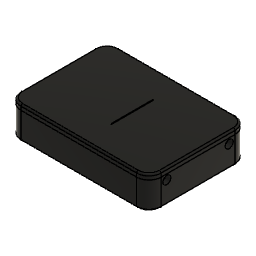
ESP-32_CAM_Box (Autodesk Fusion 360 design; units mm, degrees)
Autodesk Fusion 360 part; units mm, degrees
ref_plane "WorkPlane1" through (0, 0, -4.6) normal (0, 0, 1) x (1, 0, 0)
sketch "Sketch1" plane through (0, 0, -4.6) normal (0, 0, 1) x (1, 0, 0)
  line L0 (-20, 11.5) -> (-20, -11.5)
  arc A0 (-18, 13.5) -> (-20, 11.5) centre (-18, 11.5) ccw
  line L1 (18, 13.5) -> (-18, 13.5)
  arc A1 (20, 11.5) -> (18, 13.5) centre (18, 11.5) ccw
  line L2 (20, -11.5) -> (20, 11.5)
  arc A2 (18, -13.5) -> (20, -11.5) centre (18, -11.5) ccw
  line L3 (-18, -13.5) -> (18, -13.5)
  arc A3 (-20, -11.5) -> (-18, -13.5) centre (-18, -11.5) ccw
  arc A4 (-21.8, -11.5) -> (-18, -15.3) centre (-18, -11.5) ccw
  line L4 (-18, -15.3) -> (18, -15.3)
  arc A5 (18, -15.3) -> (21.8, -11.5) centre (18, -11.5) ccw
  line L5 (21.8, -11.5) -> (21.8, 11.5)
  arc A6 (21.8, 11.5) -> (18, 15.3) centre (18, 11.5) ccw
  line L6 (18, 15.3) -> (-18, 15.3)
  arc A7 (-18, 15.3) -> (-21.8, 11.5) centre (-18, 11.5) ccw
  line L7 (-21.8, 11.5) -> (-21.8, -11.5)
  line L8 (-20.2, 11.5) -> (-20.2, -11.5)
  arc A8 (-20.2, -11.5) -> (-18, -13.7) centre (-18, -11.5) ccw
  line L9 (-18, -13.7) -> (18, -13.7)
  arc A9 (18, -13.7) -> (20.2, -11.5) centre (18, -11.5) ccw
  line L10 (20.2, -11.5) -> (20.2, 11.5)
  arc A10 (20.2, 11.5) -> (18, 13.7) centre (18, 11.5) ccw
  line L11 (18, 13.7) -> (-18, 13.7)
  arc A11 (-18, 13.7) -> (-20.2, 11.5) centre (-18, 11.5) ccw
  dimension "d1" = 1.8
  dimension "d2" = 0.2
extrude "Extrude1" add sketch "Sketch1" along normal blind 8.4 contours L0 A0 L1 A1 L2 A2 L3 A3 | A4 L4 A5 L5 A6 L6 A7 L7 | L8 A8 L9 A9 L10 A10 L11 A11 makes body 1
shell "Shell1" thickness 1.6 removed faces 1 at (6, -5.1, 3.8) on bodies 1
sketch "Sketch3" plane through (0, 0, -3) normal (0, 0, 1) x (-1, 0, 0)
  line L0 (20.2, -11.5) -> (20.2, 11.5)
  arc A0 (20.2, 11.5) -> (18, 13.7) centre (18, 11.5) ccw
  line L1 (18, 13.7) -> (-18, 13.7)
  arc A1 (-18, 13.7) -> (-20.2, 11.5) centre (-18, 11.5) ccw
  line L2 (-20.2, 11.5) -> (-20.2, -11.5)
  arc A2 (-20.2, -11.5) -> (-18, -13.7) centre (-18, -11.5) ccw
  line L3 (-18, -13.7) -> (18, -13.7)
  arc A3 (18, -13.7) -> (20.2, -11.5) centre (18, -11.5) ccw
  line L4 (-9, -1.4583) -> (-9, -7.75)
  line L5 (-12.5, -0.8045) -> (-9.6602, -0.8045)
  line L6 (-12.5, 7.75) -> (-12.5, -0.8045)
  line L7 (-9, -7.75) -> (4.5, -7.75)
  line L8 (4.5, -7.75) -> (4.5, 7.75)
  line L9 (4.5, 7.75) -> (-12.5, 7.75)
  line L10 (-12.7, 7.95) -> (-12.7, -1.0045)
  line L11 (-12.7, -1.0045) -> (-9.5, -1.0045)
  line L12 (-9.2, -1.3) -> (-9.2, -7.95)
  line L13 (-9.2, -7.95) -> (4.7, -7.95)
  line L14 (4.7, -7.95) -> (4.7, 7.95)
  line L15 (4.7, 7.95) -> (-12.7, 7.95)
  line L16 (-9.6602, -0.8045) -> (-9, -0.8045)
  line L17 (-9, -0.8045) -> (-9, -1.4583)
  line L18 (-9.5, -1.0045) -> (-9.2, -1.0045)
  line L19 (-9.2, -1.0045) -> (-9.2, -1.3)
  line L20 (-3.08, -12.5) -> (-1.48, -12.5)
  line L21 (-3.28, -10.7) -> (-3.28, -12.3)
  line L22 (-1.48, -10.5) -> (-3.08, -10.5)
  line L23 (14.7, -12.5) -> (16.3, -12.5)
  line L24 (16.5, -12.3) -> (16.5, -10.7)
  line L25 (16.3, -10.5) -> (14.7, -10.5)
  line L26 (-3.28, 10.7) -> (-3.28, 12.3)
  line L27 (-1.48, 10.5) -> (-3.08, 10.5)
  line L28 (-3.08, 12.5) -> (-1.48, 12.5)
  line L29 (16.3, 10.5) -> (14.7, 10.5)
  line L30 (16.5, 12.3) -> (16.5, 10.7)
  line L31 (14.7, 12.5) -> (16.3, 12.5)
  line L32 (-1.48, -10.5) -> (14.7, -10.5)
  line L33 (-1.48, -12.5) -> (14.7, -12.5)
  line L34 (-3.28, -10.7) -> (-3.28, -10.5)
  line L35 (-3.28, -10.5) -> (-3.08, -10.5)
  line L36 (-3.28, -12.3) -> (-3.28, -12.5)
  line L37 (-3.28, -12.5) -> (-3.08, -12.5)
  line L38 (16.5, -10.7) -> (16.5, -10.5)
  line L39 (16.5, -10.5) -> (16.3, -10.5)
  line L40 (16.5, -12.3) -> (16.5, -12.5)
  line L41 (16.5, -12.5) -> (16.3, -12.5)
  line L42 (-1.48, 12.5) -> (14.7, 12.5)
  line L43 (14.7, 10.5) -> (-1.48, 10.5)
  line L44 (-3.08, 10.5) -> (-3.28, 10.5)
  line L45 (-3.28, 10.7) -> (-3.28, 10.5)
  line L46 (-3.28, 12.3) -> (-3.28, 12.5)
  line L47 (-3.28, 12.5) -> (-3.08, 12.5)
  line L48 (16.3, 12.5) -> (16.5, 12.5)
  line L49 (16.5, 12.5) -> (16.5, 12.3)
  line L50 (16.5, 10.7) -> (16.5, 10.5)
  line L51 (16.5, 10.5) -> (16.3, 10.5)
  line L52 (16.3, 12.7) -> (16.7, 12.7)
  line L53 (16.7, 12.7) -> (16.7, 12.3)
  line L54 (16.7, 12.3) -> (16.7, 10.7)
  line L55 (16.7, 10.7) -> (16.7, 10.3)
  line L56 (16.7, 10.3) -> (16.3, 10.3)
  line L57 (16.3, 10.3) -> (14.7, 10.3)
  line L58 (14.7, 10.3) -> (-1.48, 10.3)
  line L59 (-1.48, 10.3) -> (-3.08, 10.3)
  line L60 (-3.08, 10.3) -> (-3.48, 10.3)
  line L61 (-3.48, 10.7) -> (-3.48, 10.3)
  line L62 (-3.48, 10.7) -> (-3.48, 12.3)
  line L63 (-3.48, 12.3) -> (-3.48, 12.7)
  line L64 (-3.48, 12.7) -> (-3.08, 12.7)
  line L65 (-3.08, 12.7) -> (-1.48, 12.7)
  line L66 (-1.48, 12.7) -> (14.7, 12.7)
  line L67 (14.7, 12.7) -> (16.3, 12.7)
  line L68 (-1.48, -10.3) -> (14.7, -10.3)
  line L69 (16.3, -10.3) -> (14.7, -10.3)
  line L70 (16.7, -10.3) -> (16.3, -10.3)
  line L71 (16.7, -10.7) -> (16.7, -10.3)
  line L72 (16.7, -12.3) -> (16.7, -10.7)
  line L73 (16.7, -12.3) -> (16.7, -12.7)
  line L74 (16.7, -12.7) -> (16.3, -12.7)
  line L75 (14.7, -12.7) -> (16.3, -12.7)
  line L76 (-1.48, -12.7) -> (14.7, -12.7)
  line L77 (-3.08, -12.7) -> (-1.48, -12.7)
  line L78 (-3.48, -12.7) -> (-3.08, -12.7)
  line L79 (-3.48, -12.3) -> (-3.48, -12.7)
  line L80 (-3.48, -10.7) -> (-3.48, -12.3)
  line L81 (-3.48, -10.7) -> (-3.48, -10.3)
  line L82 (-3.48, -10.3) -> (-3.08, -10.3)
  line L83 (-1.48, -10.3) -> (-3.08, -10.3)
  line L84 (15.375, 11.825) -> (15.625, 11.825)
  arc A4 (15.825, 11.625) -> (15.625, 11.825) centre (15.625, 11.625) ccw
  line L85 (15.825, 11.625) -> (15.825, 11.375)
  arc A5 (15.375, 11.825) -> (15.175, 11.625) centre (15.375, 11.625) ccw
  line L86 (15.175, 11.375) -> (15.175, 11.625)
  arc A6 (15.175, 11.375) -> (15.375, 11.175) centre (15.375, 11.375) ccw
  line L87 (15.625, 11.175) -> (15.375, 11.175)
  arc A7 (15.625, 11.175) -> (15.825, 11.375) centre (15.625, 11.375) ccw
  line L88 (15.375, 11.925) -> (15.625, 11.925)
  arc A8 (15.925, 11.625) -> (15.625, 11.925) centre (15.625, 11.625) ccw
  line L89 (15.925, 11.625) -> (15.925, 11.375)
  arc A9 (15.625, 11.075) -> (15.925, 11.375) centre (15.625, 11.375) ccw
  line L90 (15.625, 11.075) -> (15.375, 11.075)
  arc A10 (15.075, 11.375) -> (15.375, 11.075) centre (15.375, 11.375) ccw
  line L91 (15.075, 11.375) -> (15.075, 11.625)
  arc A11 (15.375, 11.925) -> (15.075, 11.625) centre (15.375, 11.625) ccw
  circle A12 centre (17, 8.5) radius 1.1
  dimension "d12" = -0.2
  dimension "d13" = 0.2
  dimension "d16" = -0.1
  constraint coincident L5.end L16.start
  constraint parallel L5 L16
  constraint coincident L4.start L17.end
  constraint perpendicular L12 L18
  constraint perpendicular L11 L19
  constraint coincident L22.start L32.start
  constraint coincident L25.end L32.end
  constraint coincident L20.end L33.start
  constraint coincident L23.start L33.end
  constraint coincident L21.start L34.start
  constraint perpendicular L22 L34
  constraint coincident L22.end L35.end
  constraint perpendicular L21 L35
  constraint coincident L21.end L36.start
  constraint perpendicular L22 L36
  constraint coincident L20.start L37.end
  constraint perpendicular L21 L37
  constraint coincident L24.end L38.start
  constraint perpendicular L25 L38
  constraint coincident L25.start L39.end
  constraint perpendicular L38 L39
  constraint coincident L24.start L40.start
  constraint perpendicular L25 L40
  constraint coincident L23.end L41.end
  constraint coincident L28.end L42.start
  constraint coincident L31.start L42.end
  constraint coincident L29.end L43.start
  constraint coincident L27.start L43.end
  constraint coincident L27.end L44.start
  constraint perpendicular L26 L44
  constraint coincident L26.start L45.start
  constraint perpendicular L44 L45
  constraint coincident L26.end L46.start
  constraint perpendicular L28 L46
  constraint coincident L28.start L47.end
  constraint perpendicular L46 L47
  constraint coincident L31.end L48.start
  constraint perpendicular L46 L48
  constraint coincident L30.start L49.end
  constraint coincident L30.end L50.start
  constraint perpendicular L31 L50
  constraint coincident L29.start L51.end
  measures "d12" distance of L48
extrude "Extrude3" cut sketch "Sketch3" against normal blind 1.25 contours L4 L5 L6 L7 L8 L9 L16 L17 | L10 L11 L12 L13 L14 L15 L18 L19 bodies 1
extrude "Extrude4" cut sketch "Sketch3" against normal blind 0.5 contours L20 L21 L22 L23 L24 L25 L32 L33 L34 L35 L36 L37 L38 L39 L40 L41 | L26 L27 L28 L29 L30 L31 L42 L43 L44 L45 L46 L47 L48 L49 L50 L51 | L52 L53 L54 L55 L56 L57 L58 L59 L60 L61 L62 L63 L64 L65 L66 L67 | L68 L69 L70 L71 L72 L73 L74 L75 L76 L77 L78 L79 L80 L81 L82 L83 | L84 A4 L85 A5 L86 A6 L87 A7 | L88 A8 L89 A9 L90 A10 L91 A11 bodies 1
extrude "Extrude5" cut sketch "Sketch3" against normal blind 1.6 contours L84 A4 L85 A5 L86 A6 L87 A7 | L88 A8 L89 A9 L90 A10 L91 A11 bodies 1
pattern_linear "R-Pattern1" count 8 spacing 2.54 along (1, 0, 0) of "Extrude5"
mirror "Mirror1" about plane through (0, 0, 0) normal (0, 1, 0) of "Extrude5", "R-Pattern1"
sketch "Sketch4" plane through (-20.2, 0, 0) normal (1, 0, 0) x (0, 1, 0)
  line L0 (-11.5, -3) -> (11.5, -3)
  line L1 (11.5, -3) -> (11.5, 3.8)
  line L2 (11.5, 3.8) -> (-11.5, 3.8)
  line L3 (-11.5, 3.8) -> (-11.5, -3)
  line L4 (7.25, 0.5) -> (7.25, 1.8)
  arc A0 (7.25, 1.8) -> (7.05, 2) centre (7.05, 1.8) ccw
  line L5 (7.05, 2) -> (-2, 2)
  line L6 (-2.4839, 2) -> (-2, 2)
  line L7 (-2.4839, 2) -> (-4.0123, 2)
  line L8 (-4.0123, 2) -> (-4.4962, 2)
  line L9 (-4.4962, 2) -> (-7.05, 2)
  arc A1 (-7.05, 2) -> (-7.25, 1.8) centre (-7.05, 1.8) ccw
  line L10 (-7.25, 0.5) -> (-7.25, 1.8)
  line L11 (-7.25, 0.5) -> (-4.4962, 0.5)
  line L12 (-4.0123, 0.5) -> (-4.4962, 0.5)
  line L13 (-2.4839, 0.5) -> (-4.0123, 0.5)
  line L14 (-2, 0.5) -> (-2.4839, 0.5)
  line L15 (7.25, 0.5) -> (-2, 0.5)
extrude "Extrude6" cut sketch "Sketch4" against normal blind 1.6 contours L4 A0 L5 L6 L7 L8 L9 A1 L10 L11 L12 L13 L14 L15 bodies 1
extrude "Extrude7" cut sketch "Sketch3" against normal blind 1.6 contours A12 bodies 1
sketch "Sketch5" plane through (0, 0, 3.8) normal (0, 0, 1) x (-1, 0, 0)
  arc A0 (18, -13.7) -> (20.2, -11.5) centre (18, -11.5) ccw
  line L0 (18, -13.7) -> (-18, -13.7)
  arc A1 (-20.2, -11.5) -> (-18, -13.7) centre (-18, -11.5) ccw
  line L1 (-20.2, -11.5) -> (-20.2, 11.5)
  arc A2 (-18, 13.7) -> (-20.2, 11.5) centre (-18, 11.5) ccw
  line L2 (-18, 13.7) -> (18, 13.7)
  arc A3 (20.2, 11.5) -> (18, 13.7) centre (18, 11.5) ccw
  line L3 (20.2, 11.5) -> (20.2, -11.5)
  line L4 (21.8, -11.5) -> (21.8, 11.5)
  arc A4 (21.8, 11.5) -> (18, 15.3) centre (18, 11.5) ccw
  line L5 (18, 15.3) -> (-18, 15.3)
  arc A5 (-18, 15.3) -> (-21.8, 11.5) centre (-18, 11.5) ccw
  line L6 (-21.8, 11.5) -> (-21.8, -11.5)
  arc A6 (-21.8, -11.5) -> (-18, -15.3) centre (-18, -11.5) ccw
  line L7 (-18, -15.3) -> (18, -15.3)
  arc A7 (18, -15.3) -> (21.8, -11.5) centre (18, -11.5) ccw
extrude "Extrude8" add sketch "Sketch5" along normal blind 1.6 separate body contours A0 L0 A1 L1 A2 L2 A3 L3 | L4 A4 L5 A5 L6 A6 L7 A7 makes body 2
sketch "Sketch6" plane through (0, 0, 5.4) normal (0, 0, 1) x (-1, 0, 0)
  arc A0 (18, -15.3) -> (21.8, -11.5) centre (18, -11.5) ccw
  line L0 (21.8, -11.5) -> (21.8, 11.5)
  arc A1 (21.8, 11.5) -> (18, 15.3) centre (18, 11.5) ccw
  line L1 (18, 15.3) -> (-18, 15.3)
  arc A2 (-18, 15.3) -> (-21.8, 11.5) centre (-18, 11.5) ccw
  line L2 (-21.8, 11.5) -> (-21.8, -11.5)
  arc A3 (-21.8, -11.5) -> (-18, -15.3) centre (-18, -11.5) ccw
  line L3 (-18, -15.3) -> (18, -15.3)
  line L4 (-1.275, 3.0995) -> (-1.275, -3.0995)
  line L5 (-1.375, -3.0995) -> (-1.375, 3.0995)
  line L6 (-1.375, -3.0995) -> (-1.375, -6.4995)
  line L7 (-1.275, -3.0995) -> (-1.275, -6.4995)
  line L8 (-1.275, -6.4995) -> (-1.375, -6.4995)
  line L9 (-1.375, 3.0995) -> (-1.375, 6.4995)
  line L10 (-1.275, 3.0995) -> (-1.275, 6.4995)
  line L11 (-1.275, 6.4995) -> (-1.375, 6.4995)
  line L12 (-1.45, -3.0995) -> (-1.45, -6.4995)
  line L13 (-1.45, -3.0995) -> (-1.45, 3.0995)
  line L14 (-1.45, 3.0995) -> (-1.45, 6.4995)
  line L15 (-1.2, 3.0995) -> (-1.2, -3.0995)
  line L16 (-1.2, -3.0995) -> (-1.2, -6.4995)
  line L17 (-1.2, -6.4995) -> (-1.275, -6.4995)
  line L18 (-1.45, -6.4995) -> (-1.375, -6.4995)
  line L19 (-1.2, 3.0995) -> (-1.2, 6.4995)
  line L20 (-1.2, 6.4995) -> (-1.275, 6.4995)
  line L21 (-1.45, 6.4995) -> (-1.375, 6.4995)
  dimension "d31" = 3.4
  dimension "d32" = 3.4
  dimension "d33" = 3.4
  dimension "d34" = -0.075
  dimension "d35" = -0.075
  constraint coincident L4.end L7.start
  constraint parallel L4 L7
  constraint perpendicular L6 L8
  constraint coincident L5.end L9.start
  constraint parallel L5 L9
  constraint coincident L4.start L10.start
  constraint parallel L9 L10
  constraint perpendicular L9 L11
  constraint perpendicular L8 L16
  constraint perpendicular L7 L17
  constraint perpendicular L6 L18
  constraint parallel L10 L19
  constraint perpendicular L10 L20
  constraint perpendicular L9 L21
  measures "d31" distance of L5.start L6.end
  measures "d32" distance of L4.end L7.end
  measures "d33" distance of L5.end L9.end
extrude "Extrude9" cut sketch "Sketch6" against normal blind 1.6 contours L4 L7 L10 L15 L16 L17 L19 L20 | L4 L5 L6 L7 L8 L9 L10 L11 | L5 L6 L9 L12 L13 L14 L18 L21 bodies 2
sketch "Sketch7" plane through (0, 0, 3.8) normal (0, 0, -1) x (1, 0, 0)
  line L0 (1.45, -6.4995) -> (1.2, -6.4995)
  line L1 (1.2, -6.4995) -> (1.2, 6.4995)
  line L2 (1.2, 6.4995) -> (1.45, 6.4995)
  line L3 (1.45, 6.4995) -> (1.45, -6.4995)
  arc A0 (-21.8, -11.5) -> (-18, -15.3) centre (-18, -11.5) ccw
  line L4 (-18, -15.3) -> (18, -15.3)
  arc A1 (18, -15.3) -> (21.8, -11.5) centre (18, -11.5) ccw
  line L5 (21.8, -11.5) -> (21.8, 11.5)
  arc A2 (21.8, 11.5) -> (18, 15.3) centre (18, 11.5) ccw
  line L6 (18, 15.3) -> (-18, 15.3)
  arc A3 (-18, 15.3) -> (-21.8, 11.5) centre (-18, 11.5) ccw
  line L7 (-21.8, 11.5) -> (-21.8, -11.5)
  line L8 (20.2, -11.5) -> (20.2, 11.5)
  arc A4 (20.2, 11.5) -> (18, 13.7) centre (18, 11.5) ccw
  line L9 (18, 13.7) -> (-18, 13.7)
  line L10 (-20.2, 11.5) -> (-20.2, -11.5)
  arc A5 (-18, 13.7) -> (-20.2, 11.5) centre (-18, 11.5) ccw
  arc A6 (-20.2, -11.5) -> (-18, -13.7) centre (-18, -11.5) ccw
  line L11 (-18, -13.7) -> (18, -13.7)
  arc A7 (18, -13.7) -> (20.2, -11.5) centre (18, -11.5) ccw
  line L12 (-20.2, -11.5) -> (-18.6, -11.5)
  line L13 (-18.6, -11.5) -> (-18.6, -7.9)
  line L14 (-18.6, -7.9) -> (-20.2, -7.9)
  line L15 (-20.2, -7.9) -> (-20.2, -11.5)
  dimension "d38" = 1.6
  dimension "d39" = 3.6
  constraint horizontal L12
  constraint vertical L13
  constraint horizontal L14
  constraint vertical L15
  constraint coincident L10.end A6.start
  measures "d38" distance of L10.end L12.end
  measures "d39" distance of L10.end L14.end
extrude "Extrude10" add sketch "Sketch7" along normal blind 3.3 contours L10 L12 L13 L14 L15 bodies 2
sketch "Sketch8" plane through (-20.2, 0, 0) normal (-1, 0, 0) x (0, -1, 0)
  line L0 (-7.9, 3.8) -> (-11.5, 3.8)
  line L1 (-11.5, 3.8) -> (-11.5, 0.5)
  line L2 (-11.5, 0.5) -> (-7.9, 0.5)
  line L3 (-7.9, 0.5) -> (-7.9, 3.8)
  circle A0 centre (-9.7, 2.15) radius 0.65
  point P0 (-9.7, 2.15)
  dimension "d42" = 1.3
  constraint coincident P0 A0.centre
  measures "d42" diameter of A0
extrude "Extrude11" cut sketch "Sketch8" against normal blind 1.6 contours A0 bodies 2
fillet "Fillet1" radius 1 2 edges at (-19.4, 11.5, 0.5) (-19.4, 7.9, 0.5) on bodies 2
sketch "Sketch9" plane through (-21.8, 0, 0) normal (-1, 0, 0) x (0, -1, 0)
  line L0 (-7.05, 2) -> (7.05, 2)
  arc A0 (7.25, 1.8) -> (7.05, 2) centre (7.05, 1.8) ccw
  line L1 (7.25, 1.8) -> (7.25, 0.5)
  line L2 (7.25, 0.5) -> (-7.25, 0.5)
  line L3 (-7.25, 0.5) -> (-7.25, 1.8)
  arc A1 (-7.05, 2) -> (-7.25, 1.8) centre (-7.05, 1.8) ccw
  line L4 (-11.5, -4.6) -> (11.5, -4.6)
  line L5 (11.5, -4.6) -> (11.5, 3.8)
  line L6 (11.5, 3.8) -> (-11.5, 3.8)
  line L7 (-11.5, 3.8) -> (-11.5, -4.6)
  circle A2 centre (-9.7, 2.15) radius 0.65
  circle A3 centre (-9.7, 2.15) radius 1.25
  dimension "d49" = 0.6
extrude "Extrude12" cut sketch "Sketch9" against normal blind 1.6 contours A2 | A3 bodies 1
mirror "Mirror4" about plane through (0, 0, 0) normal (1, 0, 0) of "Extrude10", "Extrude11", "Fillet1", "Extrude12"
mirror "Mirror5" about plane through (0, 0, 0) normal (0, 1, 0) of "Extrude10", "Extrude11", "Fillet1", "Extrude12", "Mirror4"
fillet "Fillet2" radius 0.5 16 edges at (0, 15.3, -4.6) (-20.687, 14.187, -4.6) (-21.8, 0, -4.6) (-20.687, -14.187, -4.6) (0, -15.3, -4.6) (20.687, -14.187, -4.6) (21.8, 0, -4.6) (20.687, 14.187, -4.6) (0, 15.3, 5.4) (-20.687, 14.187, 5.4) (-21.8, 0, 5.4) (-20.687, -14.187, 5.4) (0, -15.3, 5.4) (20.687, -14.187, 5.4) (21.8, 0, 5.4) (20.687, 14.187, 5.4) on bodies 1 2
named bodies: "Case", "Cap"
